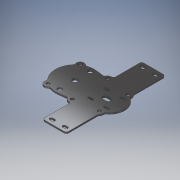
# Autodesk Inventor part: SIDE REDUCTION PLATE II
Saved by Autodesk Inventor 2017 (Build 210142000, 142)
## iProperties
Part Number: SIDE REDUCTION PLATE II
Material: Genérico
Document SubType Name: Modeling
Designer: Cristian
Density: 1 g/cm^3
Appearance: Valor por defecto
Author: Cristian
Autodesk Inventor part; units mm, degrees
ref_plane "XZ Plane" through (0, 0, 0) normal (0, 1, 0) x (-1, 0, 0)
ref_plane "XY Plane" through (0, 0, 0) normal (0, 0, 1) x (1, 0, 0)
sketch "Boceto1" plane through (0, 0, 0) normal (0, 0, 1) x (1, 0, 0)
  circle A0 centre (0, 0) radius 57.15
  circle A1 centre (101.6, 0) radius 44.45
  circle A2 centre (-31.75, 47.519) radius 11.1125
  circle A3 centre (-31.75, -47.519) radius 11.1125
  circle A4 centre (114.3, 42.5971) radius 11.1125
  circle A5 centre (114.3, -42.5971) radius 11.1125
  line L0 (7.1437, 56.7018) -> (107.1562, 44.1014)
  circle A6 centre (44.45, 52.0016) radius 11.1125
  line L1 (7.1437, -56.7018) -> (107.1562, -44.1014)
  circle A7 centre (44.45, -52.0016) radius 11.1125
  dimension "d0" = 114.3
  dimension "d1" = 88.9
  dimension "d2" = 203.2
  dimension "d3" = 22.225
  dimension "d4" = 22.225
  dimension "d7" = 22.225
  dimension "d8" = 22.225
  dimension "d11" = 22.225
  dimension "d13" = 0
  dimension "d14" = 22.225
  dimension "d35" = 31.75
  dimension "d36" = 31.75
  dimension "d37" = 44.45
  dimension "d38" = 44.45
  dimension "d39" = 12.7
  dimension "d40" = 12.7
  constraints: 8 centre point, 8 point on circle, 4 end point, 4 tangent, 2 point on line, 1 coincident
  measures "d0" diameter of A0
  measures "d1" diameter of A1
  measures "d3" diameter of A2
  measures "d4" diameter of A3
  measures "d7" diameter of A4
  measures "d8" diameter of A5
  measures "d11" diameter of A6
  measures "d13" vertical distance of point (0, 0) A1.centre
  measures "d14" diameter of A7
  measures "d35" horizontal distance of A0.centre A3.centre
  measures "d36" horizontal distance of A0.centre A2.centre
  measures "d37" horizontal distance of point (0, 0) A7.centre
  measures "d38" horizontal distance of point (0, 0) A6.centre
  measures "d39" horizontal distance of A1.centre A5.centre
  measures "d40" horizontal distance of A1.centre A4.centre
extrude "Extrusión1" add sketch "Boceto1" along normal blind 4.445
ref_plane "Plano de trabajo1" through (50.8, 0, 0) normal (1, 0, 0) x (0, 1, 0)
sketch "Boceto3" plane through (50.8, 0, 0) normal (1, 0, 0) x (0, 1, 0)
  line L0 (0, 0) -> (0, 4.445)
  line L1 (-52.7651, 4.445) -> (-56.7018, 4.445) projected
  line L2 (0, 4.445) -> (69.85, 4.445)
  line L3 (69.85, 4.445) -> (69.85, 4.445)
  line L4 (69.85, 4.445) -> (146.05, 4.445)
  line L5 (146.05, 4.445) -> (146.05, 0)
  line L6 (146.05, 0) -> (74.295, 0)
  line L7 (74.295, 0) -> (74.295, 0)
  line L8 (74.295, 0) -> (0, 0)
  point P0 (37.2916, 4.445)
  point P1 (-37.2916, 4.445)
  dimension "d28" = 4.445
  dimension "d29" = 4.445
  dimension "d30" = 69.85
  dimension "d31" = 4.445
  dimension "d32" = 146.05
  constraints: 16 end point, 6 perpendicular, 1 horizontal, 1 point on line
  measures "d28" distance between parallel lines of L7 L3
  measures "d29" distance between parallel lines of L4 L6
  measures "d30" distance of L0.end L2.end
  measures "d31" distance between parallel lines of L4 L8
  measures "d32" distance between parallel lines of L0 L5
extrude "Extrusión3" add sketch "Boceto3" along normal blind 69.85
fillet "Empalme5" radius 6.35 2 edges at (120.65, 146.05, 2.2225) (50.8, 146.05, 2.2225)
mirror "Simetría1" about plane through (0, 0, 0) normal (0, 1, 0) of "Extrusión3", "Empalme5"
sketch "Boceto2" plane through (0, 0, 4.445) normal (0, 0, 1) x (1, 0, 0)
  arc A0 (-21.9537, 52.7651) -> (-40.3458, 40.4764) centre (-31.75, 47.519) ccw projected
  circle A1 centre (-31.75, 47.519) radius 4.7625
  arc A2 (-40.3458, -40.4764) -> (-21.9537, -52.7651) centre (-31.75, -47.519) ccw projected
  circle A3 centre (-31.75, -47.519) radius 4.7625
  arc A4 (33.4247, -53.3907) -> (55.4753, -50.6125) centre (44.45, -52.0016) ccw projected
  circle A5 centre (44.45, -52.0016) radius 4.7625
  arc A6 (55.4753, 50.6125) -> (33.4247, 53.3907) centre (44.45, 52.0016) ccw projected
  circle A7 centre (44.45, 52.0016) radius 4.7625
  arc A8 (124.4689, 38.1158) -> (103.3657, 44.5789) centre (114.3, 42.5971) ccw projected
  circle A9 centre (114.3, 42.5971) radius 4.7625
  arc A10 (103.3657, -44.5789) -> (124.4689, -38.1158) centre (114.3, -42.5971) ccw projected
  circle A11 centre (114.3, -42.5971) radius 4.7625
  point P0 (0, 0)
  dimension "d18" = 9.525
  dimension "d19" = 9.525
  dimension "d20" = 9.525
  dimension "d21" = 9.525
  dimension "d22" = 9.525
  dimension "d23" = 9.525
  constraints: 6 centre point, 6 coincident
  measures "d18" diameter of A1
  measures "d19" diameter of A3
  measures "d20" diameter of A5
  measures "d21" diameter of A7
  measures "d22" diameter of A9
  measures "d23" diameter of A11
extrude "Extrusión2" cut sketch "Boceto2" against normal up to surface (4.445 mm away)
fillet "Empalme6" radius 6.35 12 edges at (124.4689, 38.1158, 2.2225) (120.65, 51.7166, 2.2225) (-40.3458, 40.4764, 2.2225) (-21.9537, 52.7651, 2.2225) (124.4689, -38.1158, 2.2225) (120.65, -51.7166, 2.2225) (-21.9537, -52.7651, 2.2225) (-40.3458, -40.4764, 2.2225) (33.4247, -53.3907, 2.2225) (50.8, -61.1211, 2.2225) (50.8, 61.1211, 2.2225) (33.4247, 53.3907, 2.2225)
sketch "Boceto5" plane through (0, 0, 4.445) normal (0, 0, 1) x (1, 0, 0)
  circle A0 centre (0, 0) radius 7.1437
  line L0 (0, 0) -> (0, 45)
  line L1 (0, 0) -> (0, -45)
  circle A1 centre (0, 45) radius 6.35
  circle A2 centre (0, -45) radius 6.35
  dimension "d58" = 14.2875
  dimension "d59" = 45
  dimension "d60" = 45
  dimension "d61" = 12.7
  dimension "d62" = 12.7
  constraints: 4 end point, 3 centre point, 3 coincident, 2 vertical
  measures "d58" diameter of A0
  measures "d59" distance of L0.start L0.end
  measures "d60" distance of L0.start L1.end
  measures "d61" diameter of A1
  measures "d62" diameter of A2
extrude "Extrusión5" cut sketch "Boceto5" against normal up to surface (4.445 mm away)
sketch "Boceto6" plane through (0, 0, 4.445) normal (0, 0, 1) x (1, 0, 0)
  circle A0 centre (93.4212, 0) radius 6.35
  circle A1 centre (88.2618, 0) radius 6.35
  circle A2 centre (98.5806, 0) radius 6.35
  line L0 (88.2618, 6.35) -> (98.5806, 6.35)
  line L1 (98.5806, -6.35) -> (88.2618, -6.35)
  line L2 (69.6712, 23.75) -> (117.1712, 23.75)
  line L3 (117.1712, 23.75) -> (117.1712, -23.75)
  line L4 (117.1712, -23.75) -> (69.6712, -23.75)
  line L5 (69.6712, -23.75) -> (69.6712, 23.75)
  circle A3 centre (74.8306, 23.75) radius 2.7781
  circle A4 centre (64.5118, 23.75) radius 2.7781
  line L6 (74.8306, 26.5281) -> (64.5118, 26.5281)
  line L7 (64.5118, 20.9719) -> (74.8306, 20.9719)
  circle A5 centre (74.8306, -23.75) radius 2.7781
  circle A6 centre (64.5118, -23.75) radius 2.7781
  line L8 (64.5118, -20.9719) -> (74.8306, -20.9719)
  line L9 (74.8306, -26.5281) -> (64.5118, -26.5281)
  circle A7 centre (112.0118, -23.75) radius 2.7781
  circle A8 centre (122.3306, -23.75) radius 2.7781
  line L10 (112.0118, -20.9719) -> (122.3306, -20.9719)
  line L11 (112.0118, -26.5281) -> (122.3306, -26.5281)
  circle A9 centre (112.0118, 23.75) radius 2.7781
  circle A10 centre (122.3306, 23.75) radius 2.7781
  line L12 (112.0118, 26.5281) -> (122.3306, 26.5281)
  line L13 (112.0118, 20.9719) -> (122.3306, 20.9719)
  point P0 (0, 0)
  dimension "d65" = 12.7
  dimension "d66" = 0
  dimension "d67" = 93.4212
  dimension "d68" = 12.7
  dimension "d69" = 12.7
  dimension "d70" = 5.1594
  dimension "d71" = 5.1594
  dimension "d72" = 47.5
  dimension "d73" = 47.5
  dimension "d74" = 23.75
  dimension "d75" = 23.75
  dimension "d76" = 5.5563
  dimension "d77" = 5.5563
  dimension "d78" = 5.1594
  dimension "d79" = 5.1594
  dimension "d80" = 0
  dimension "d81" = 5.5563
  dimension "d82" = 5.5563
  dimension "d83" = 5.1594
  dimension "d84" = 5.1594
  dimension "d85" = 0
  dimension "d86" = 0
  dimension "d87" = 5.5563
  dimension "d88" = 5.5563
  dimension "d89" = 5.1594
  dimension "d90" = 5.1594
  dimension "d91" = 0
  dimension "d92" = 5.5563
  dimension "d93" = 5.5563
  dimension "d94" = 5.1594
  dimension "d95" = 5.1594
  dimension "d96" = 0
  constraints: 28 end point, 20 point on circle, 20 tangent, 11 centre point, 4 point on line, 2 horizontal, 2 parallel, 1 perpendicular
  measures "d65" diameter of A0
  measures "d66" vertical distance of point (0, 0) A0.centre
  measures "d67" distance of point (0, 0) A0.centre
  measures "d68" diameter of A1
  measures "d69" diameter of A2
  measures "d70" distance of A0.centre A1.centre
  measures "d71" distance of A0.centre A2.centre
  measures "d72" distance of L2.start L2.end
  measures "d73" distance of L2.end L3.end
  measures "d74" distance from line of A0.centre L3
  measures "d75" distance from line of L2 A0.centre
  measures "d76" diameter of A3
  measures "d77" diameter of A4
  measures "d78" distance of A4.centre L2.start
  measures "d79" distance of L2.start A3.centre
  measures "d80" vertical distance of A3.centre A4.centre
  measures "d81" diameter of A5
  measures "d82" diameter of A6
  measures "d83" distance of L4.end A5.centre
  measures "d84" distance of L4.end A6.centre
  measures "d85" distance from line of L4 A6.centre
  measures "d86" vertical distance of A0.centre A2.centre
  measures "d87" diameter of A7
  measures "d88" diameter of A8
  measures "d89" distance of L3.end A7.centre
  measures "d90" distance of L3.end A8.centre
  measures "d91" vertical distance of A7.centre A8.centre
  measures "d92" diameter of A9
  measures "d93" diameter of A10
  measures "d94" distance of L2.end A9.centre
  measures "d95" distance of A10.centre L2.end
  measures "d96" vertical distance of A9.centre A10.centre
extrude "Extrusión6" cut sketch "Boceto6" against normal up to next contours A0 A2 A1 | A0 A2 | A2 A1 A0 | A0 L0 A2 | A2 L1 A0 | A0 A1 A2 | A0 A1 L0 | A2 A1 A0 | A1 A2 | L1 A1 A0 | A0 A1 | A9 L12 A10 L13 L3 L2 | A9 L2 | L2 A9 | L2 L3 L13 A9 | A3 L2 | L2 A3 | A10 | L10 A8 L11 A7 L4 L3 | L3 L4 A7 L10 | A3 L7 L5 L2 | L2 L5 L7 A4 L6 A3 | A7 L4 | A8 | A4 | A7 L4 | L8 A5 L4 L5 | L5 L4 A5 L9 A6 L8 | A5 L4 | L4 A5 | A6
sketch "Boceto7" plane through (0, 0, 4.445) normal (0, 0, 1) x (1, 0, 0)
  circle A0 centre (104.775, 133.35) radius 4.3656
  line L0 (120.65, 139.7) -> (120.65, 54.5825) projected
  line L1 (57.15, 146.05) -> (114.3, 146.05) projected
  circle A1 centre (101.4016, 133.35) radius 4.3656
  circle A2 centre (108.1484, 133.35) radius 4.3656
  line L2 (108.1484, 128.9844) -> (101.4016, 128.9844)
  line L3 (108.1484, 137.7156) -> (101.4016, 137.7156)
  circle A3 centre (66.675, 133.35) radius 4.3656
  line L4 (50.8, 69.4641) -> (50.8, 139.7) projected
  circle A4 centre (63.3016, 133.35) radius 4.3656
  circle A5 centre (70.0484, 133.35) radius 4.3656
  line L5 (70.0484, 128.9844) -> (63.3016, 128.9844)
  line L6 (70.0484, 137.7156) -> (63.3016, 137.7156)
  point P0 (0, 0)
  dimension "d99" = 8.7312
  dimension "d101" = 15.875
  dimension "d104" = 8.7312
  dimension "d105" = 8.7312
  dimension "d106" = 12.7
  dimension "d107" = 0
  dimension "d108" = 0
  dimension "d110" = 3.3734
  dimension "d111" = 3.3734
  dimension "d112" = 8.7312
  dimension "d113" = 12.7
  dimension "d114" = 15.875
  dimension "d115" = 8.7312
  dimension "d116" = 8.7312
  dimension "d117" = 0
  dimension "d118" = 0
  dimension "d119" = 3.3734
  dimension "d120" = 3.3734
  constraints: 8 end point, 8 point on circle, 8 tangent, 6 centre point
  measures "d99" diameter of A0
  measures "d101" distance from line of L0 A0.centre
  measures "d104" diameter of A1
  measures "d105" diameter of A2
  measures "d106" distance from line of A0.centre L1
  measures "d107" vertical distance of A0.centre A1.centre
  measures "d108" vertical distance of A0.centre A2.centre
  measures "d110" distance of A2.centre A0.centre
  measures "d111" distance of A0.centre A1.centre
  measures "d112" diameter of A3
  measures "d113" distance from line of L1 A3.centre
  measures "d114" distance from line of L4 A3.centre
  measures "d115" diameter of A4
  measures "d116" diameter of A5
  measures "d117" vertical distance of A3.centre A5.centre
  measures "d118" vertical distance of A3.centre A4.centre
  measures "d119" distance of A3.centre A5.centre
  measures "d120" distance of A4.centre A3.centre
extrude "Extrusión7" cut sketch "Boceto7" against normal up to next
mirror "Simetría2" about plane through (0, 0, 0) normal (0, 1, 0) of "Extrusión7"
equation "\"d16\" = t"
equation "\"d28\" = t"
equation "\"d29\" = t"
equation "\"d18\" = Q"
equation "\"d19\" = Q"
equation "\"d20\" = Q"
equation "\"d21\" = Q"
equation "\"d22\" = Q"
equation "\"d23\" = Q"
equation "\"d58\" = DF"
equation "\"d59\" = 0.5 * JF"
equation "\"d60\" = 0.5 * JF"
equation "\"d61\" = NF"
equation "\"d62\" = NF"
equation "\"d65\" = DM"
equation "\"d67\" = CM"
equation "\"d68\" = DM"
equation "\"d69\" = DM"
equation "\"d72\" = BM"
equation "\"d73\" = BM"
equation "\"d74\" = 0.5 * BM"
equation "\"d75\" = 0.5 * BM"
equation "\"d76\" = NM"
equation "\"d77\" = NM"
equation "\"d81\" = NM"
equation "\"d82\" = NM"
equation "\"d87\" = NM"
equation "\"d88\" = NM"
equation "\"d92\" = NM"
equation "\"d93\" = NM"
equation "\"d99\" = DH"
equation "\"d104\" = DH"
equation "\"d105\" = DH"
equation "\"d112\" = DH"
equation "\"d115\" = DH"
equation "\"d116\" = DH"
equation "\"t\" = 4.445"
equation "\"Q\" = 9.525"
equation "\"DF\" = 14.2875"
equation "\"NF\" = 12.7"
equation "\"DH\" = 8.73125"
equation "\"DM\" = 12.7"
equation "\"NM\" = 5.55625"
equation "\"CM\" = 93.4212"
equation "\"AM\" = 56"
equation "\"BM\" = 47.5"
equation "\"JF\" = 90"
